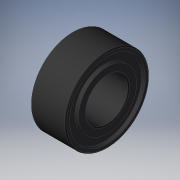
# Autodesk Inventor part: B673ZZ
Saved by Autodesk Inventor 2019 (Build 230136000, 136)
## iProperties
Created: 2023-12-09
Part Number: B673ZZ
Material: Generic
Catalog Web Link: www.cadenas.de
Description: B6 _ _ ZZ, B6 _ _ AZZ, SB6 _ _ ZZ, SB6 _ _ AZZ, BR _ _ ZZ, SBR _ _ ZZ-Small Ball Bearings - Double Shield Type
Vendor: MISUMI
Document SubType Name: Modeling
Designer: psAdmin
Manufacturer: MISUMI
Mass: 0.0481551 g
Surface Area: 1.26457 cm^2
Volume: 0.0481551 cm^3
Density: 1 g/cm^3
Appearance: PSOLRGB-175-175-175
Category: PARTsolutions
Company: MISUMI
Title: B673ZZ
Author: Cadenas PARTsolutions
Comments: Small Ball Bearings - Double Shield Type
PSOL_IDENT_0: {$CADENAS_DATA/23d-libs/misumi/metric/12_bearing_holders/sb685zz.prj},218 {VTYP=3D},{NB=B673ZZ},{LIN
PSOL_IDENT_1: A=B673ZZ},{NN=B6 _ _ ZZ, B6 _ _ AZZ, SB6 _ _ ZZ, SB6 _ _ AZZ, BR _ _ ZZ, SBR _ _ ZZ},{DATE=07.06.202
PSOL_IDENT_2: 1 10:18:38},{GEOMDATE=23.07.2013 00:00:00},{VERSION=},{LINEID=10},{WBVAR=MAT},{WBNUMERIC=}  {NB=B673
PSOL_IDENT_3: ZZ},{LINA=B673ZZ},{KT=DUMMY},{PN=B673ZZ},{MAT=},{BN=673ZZ},{DD=3.0},{A=1.9900},{BB=0.300},{C=0.575},
PSOL_IDENT_4: {D=6},{B=2.5},{RR=0.08},{CR=242},{COR=94},{CRS=242},{CRSS=178},{CORS=94},{CORSS=59},{DS=3.60},{DDHH=
PSOL_IDENT_5: 5.40},{R=0.08},{MASS=0.2},{X=0},{BN2=B673ZZ}
NB: B673ZZ
NN: B6 _ _ ZZ, B6 _ _ AZZ, SB6 _ _ ZZ, SB6 _ _ AZZ, BR _ _ ZZ, SBR _ _ ZZ
NT: Small Ball Bearings - Double Shield Type
NBSYN: $PN.
LINA: B673ZZ
CATALOG: Misumi
PN: B673ZZ
MAT: 52100 Bearing Steel
BN: 673ZZ
DD: 3
D: 6
B: 2.5
RR: 0.08
CR: 242
COR: 94
DS: 3.6
DDHH: 5.4
R: 0.08
MASS: 0.2
X: 0
SUPPLIER: MISUMI
ARTICLENO: B673ZZ
BOMINFO: B673ZZ
CREATOR: CADENAS GmbH
Autodesk Inventor part; units mm, degrees
sketch "Sketch_1" plane through (0, 0, 0) normal (0, 0, 1) x (1, 0, 0)
  line L0 (2.42, 0) -> (0.08, 0)
  arc A0 (0, 1.58) -> (0.08, 1.5) centre (0.08, 1.58) ccw
  line L1 (0.08, 1.5) -> (2.42, 1.5)
  arc A1 (2.42, 1.5) -> (2.5, 1.58) centre (2.42, 1.58) ccw
  line L2 (2.5, 1.58) -> (2.5, 2.075)
  line L3 (2.5, 2.075) -> (2.245, 2.075)
  line L4 (2.245, 2.075) -> (2.245, 2.7)
  line L5 (2.245, 2.7) -> (2.5, 2.7)
  line L6 (2.5, 2.7) -> (2.5, 2.92)
  arc A2 (2.5, 2.92) -> (2.42, 3) centre (2.42, 2.92) ccw
  line L7 (2.42, 3) -> (0.08, 3)
  arc A3 (0.08, 3) -> (0, 2.92) centre (0.08, 2.92) ccw
  line L8 (0, 2.92) -> (0, 2.7)
  line L9 (0, 2.7) -> (0.255, 2.7)
  line L10 (0.255, 2.7) -> (0.255, 2.075)
  line L11 (0.255, 2.075) -> (0, 2.075)
  line L12 (0, 2.075) -> (0, 1.58)
  constraints: 26 end point, 8 point on circle, 4 centre point
revolve "Revolution1" add sketch "Sketch_1" angle 360 about axis through (2.42, 0, 0) along (1, 0, 0)
ref_plane "to_housing_XY" through (0, 0, 0) normal (1, 0, 0) x (0, 0, -1)
ref_plane "to_housing_YZ" through (0, 0, 0) normal (0, 0, -1) x (0, 1, 0)
ref_plane "to_housing_ZX" through (0, 0, 0) normal (0, 1, 0) x (1, 0, 0)
ref_plane "to_housing_center_XY" through (1.25, 0, 0) normal (1, 0, 0) x (0, 0, -1)
ref_plane "to_housing_center_YZ" through (1.25, 0, 0) normal (0, 0, -1) x (0, 1, 0)
ref_plane "to_housing_center_ZX" through (1.25, 0, 0) normal (0, 1, 0) x (1, 0, 0)
body "Solid1"
